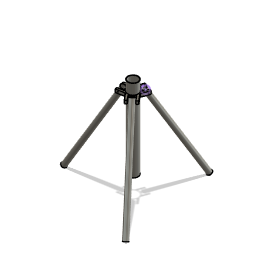
OpenTripod v8 (Autodesk Fusion 360 design; units mm, degrees)
Autodesk Fusion 360 part; units mm, degrees
note: some values were not read from the file. Set by a fixed rule: which sketch regions a step uses.
sketch "Sketch4" plane through (0, 0, 0) normal (0, 1, 0) x (1, 0, 0)
  circle A0 centre (0, 0) radius 25
  circle A1 centre (0, 0) radius 23
  dimension "d26" = 50
  dimension "d27" = 46
  constraint coincident A0.centre A1.centre
  constraint concentric A0 A1
  measures "d26" diameter of A0
  measures "d27" diameter of A1
extrude "Extrude6" add sketch "Sketch4" along normal blind 1000 makes body 1
sketch "Sketch1" plane through (0, 0, 0) normal (0, 1, 0) x (1, 0, 0)
  circle A0 centre (0, 0) radius 50
  circle A1 centre (0, 0) radius 47.5
  dimension "d1" = 100
  dimension "d2" = 95
  constraint coincident A0.centre A1.centre
  constraint concentric A0 A1
  measures "d1" diameter of A0
  measures "d2" diameter of A1
extrude "Extrude1" add sketch "Sketch1" along normal blind 800 separate body makes body 2
sketch "Sketch2" plane through (0, 800, 0) normal (0, 1, 0) x (-1, 0, 0)
  circle A0 centre (0, 0) radius 47.5
  circle A1 centre (0, 0) radius 50
  circle A2 centre (0, 0) radius 51
  circle A3 centre (0, 0) radius 60
  line L0 (0, 0) -> (-51, 0) construction
  line L1 (-51, 0) -> (-60, 0)
  line L2 (0, 0) -> (59.0885, 10.4189) construction
  line L3 (0, 0) -> (60, 0) construction
  line L4 (59.0885, 10.4189) -> (93.5567, 16.4966) construction
  circle A4 centre (93.5567, 16.4966) radius 25
  line L5 (93.5567, 16.4966) -> (89.2155, 41.1168) construction
  line L6 (89.2155, 41.1168) -> (88.3473, 46.0408) construction
  line L7 (88.3473, 46.0408) -> (45.9627, 38.5673)
  line L8 (88.3473, 46.0408) -> (108.0434, 49.5138)
  line L9 (108.0434, 49.5138) -> (104.5705, 69.2099)
  line L10 (104.5705, 69.2099) -> (23.98, 54.9996)
  line L11 (98.7662, -13.0477) -> (56.3816, -20.5212)
  line L12 (121.9353, -29.2708) -> (41.3448, -43.4811)
  line L13 (98.7662, -13.0477) -> (118.4623, -9.5747)
  line L14 (118.4623, -9.5747) -> (121.9353, -29.2708)
  line L15 (-38.0835, 92.0579) -> (-10.4189, 59.0885)
  line L16 (-38.0835, 92.0579) -> (-50.9392, 107.3787)
  line L17 (-50.9392, 107.3787) -> (-35.6184, 120.2345)
  line L18 (-35.6184, 120.2345) -> (16.9834, 57.5462)
  line L19 (-84.0462, 53.4906) -> (-56.3816, 20.5212)
  line L20 (-84.0462, 53.4906) -> (-96.9019, 68.8115)
  line L21 (-96.9019, 68.8115) -> (-112.2228, 55.9557)
  line L22 (-112.2228, 55.9557) -> (-59.6211, -6.7326)
  line L23 (-60.6827, -79.0102) -> (-45.9627, -38.5673)
  line L24 (-60.6827, -79.0102) -> (-67.5231, -97.804)
  line L25 (-67.5231, -97.804) -> (-86.3169, -90.9636)
  line L26 (-86.3169, -90.9636) -> (-58.3282, -14.0651)
  line L27 (-4.3011, -99.5314) -> (10.4189, -59.0885)
  line L28 (-4.3011, -99.5314) -> (-11.1415, -118.3253)
  line L29 (-11.1415, -118.3253) -> (7.6523, -125.1657)
  line L30 (7.6523, -125.1657) -> (35.6411, -48.2671)
  dimension "d7" = 102
  dimension "d8" = 120
  dimension "d24" = 10
  dimension "d30" = 35
  dimension "d31" = 50
  dimension "d32" = 5
  dimension "d33" = 20
  dimension "d34" = 20
  dimension "d36" = 360
  constraint coincident A0.centre A1.centre
  constraint concentric A2 A3
  constraint coincident A2 L0.end
  constraint horizontal L0
  constraint coincident A3 L1.end
  constraint parallel L0 L1
  constraint horizontal L3
  constraint coincident A3 L2.end
  constraint parallel L2 L4
  constraint coincident L4.end A4.centre
  constraint coincident A4 L5.end
  constraint perpendicular L4 L5
  constraint parallel L5 L6
  constraint coincident A3 L7.end
  constraint parallel L4 L7
  constraint perpendicular L6 L8
  constraint perpendicular L8 L9
  constraint coincident A3 L10.end
  constraint perpendicular L9 L10
  constraint symmetric L4 L6.end L11.start
  constraint symmetric L4 L7.end L11.end
  constraint symmetric L4 L8.end L13.end
  constraint symmetric L4 L9.end L12.start
  constraint symmetric L4 L10.end L12.end
  measures "d7" diameter of A2
  measures "d8" diameter of A3
  measures "d24" angle of L2 L3
  measures "d30" distance of L2.end L4.end
  measures "d31" diameter of A4
  measures "d32" distance of L5.end L6.end
  measures "d33" distance of L6.end L8.end
  measures "d34" distance of L8.end L9.end
extrude "Extrude2" add sketch "Sketch2" against normal blind 30 separate body contours A3 | A3 L7 L8 L9 L10 | A3 L11 L12 L13 L14 | A3 L15 L16 L17 L18 | A3 L27 L28 L29 L30 | A3 L19 L20 L21 L22 | A3 L23 L24 L25 L26 makes body 3
sketch "Sketch5" plane through (-8.6824, 0, -49.2404) normal (-0.173648, 0, -0.984808) x (-0.984808, 0, 0.173648)
  line L0 (115, 800) -> (33.1662, 800)
  line L1 (33.1662, 800) -> (33.1662, 770)
  line L2 (33.1662, 770) -> (115, 770)
  line L3 (115, 770) -> (115, 800)
  line L4 (115, 800) -> (80, 770) construction
  circle A0 centre (94.9882, 782.8471) radius 4.1
  dimension "d37" = 8.2
  constraint coincident L0.start L3.end
  constraint coincident L2 L4.end
  constraint coincident L4 A0.centre
  measures "d37" diameter of A0
extrude "Extrude7" cut sketch "Sketch5" against normal blind 100 contours A0 bodies 3
pattern_circular "C-Pattern1" count 3 over 360 about axis through (0, 800, 0) along (0, -1, 0) of "Extrude7"
ref_plane "WorkPlane1" through (28.5521, 785, -78.4463) normal (-0.939693, 0, -0.34202) x (0.34202, 0, -0.939693)
sketch "Sketch6" plane through (0, 0, 0) normal (-0.939693, 0, -0.34202) x (0.34202, 0, -0.939693)
  circle A0 centre (94.9882, -782.8471) radius 4.1
move_body "Move1" bodies 1 to x (1, 0, 0) y (0, 1, 0) z (0, 0, 1) at (32.4879, -217.1529, -89.2597)
move_body "Move2" bodies 1 to x (1, 0, 0) y (0, 1, 0) z (0, 0, 1) at (0, 25, 0)
move_body "Move3" bodies 1 to x (0.984328, 0.17101, 0.043059) y (-0.17101, 0.866025, 0.469846) z (0.043059, -0.469846, 0.881697) at (138.2273, 57.3875, -379.7763)
pattern_circular "C-Pattern2" count 3 over 360 about axis through (0, 1.75, 0) along (0, 1, 0) of bodies 1 makes body 4 at (-251.7543, 521.8007, 66.6853) makes body 5 at (148.9374, 521.2461, 212.5381)
move_body "Move4" bodies 2 to x (1, 0, 0) y (0, 1, 0) z (0, 0, 1) at (0, 100, 0)
equation "Tolerance = 0.2 mm"
equation "CenterPoleSize = 100 mm"
equation "d7 = CenterPoleSize + 2 mm"
equation "LegDiameter = 50 mm"
equation "d26 = LegDiameter"
equation "d27 = LegDiameter - 4 mm"
equation "d30 = LegDiameter / 2 + 10 mm"
equation "d31 = LegDiameter"
equation "d37 = 8 mm + Tolerance"
equation "d43 = LegDiameter / 2"
